Autodesk Inventor part; units mm, degrees
(part 8 of 13)
  line L3379 (11.7489, 33.1395) -> (11.9957, 33.1395) construction
  line L3380 (11.9957, 33.1395) -> (12.1959, 33.3398) construction
  line L3381 (12.1959, 33.3398) -> (12.1959, 33.5866) construction
  spline S1052 degree 3 poles (14.75, 33.5866) (14.75, 33.8334) (14.5498, 34.0334) (14.303, 34.0334) knots 0 0 0 0 1 1 1 1
  line L3382 (14.75, 33.5866) -> (14.75, 33.8334) construction
  line L3383 (14.75, 33.8334) -> (14.5498, 34.0334) construction
  line L3384 (14.5498, 34.0334) -> (14.303, 34.0334) construction
  spline S1053 degree 3 poles (14.303, 34.0334) (14.0562, 34.0334) (13.8561, 33.8334) (13.8561, 33.5866) knots 0 0 0 0 1 1 1 1
  line L3385 (14.303, 34.0334) -> (14.0562, 34.0334) construction
  line L3386 (14.0562, 34.0334) -> (13.8561, 33.8334) construction
  line L3387 (13.8561, 33.8334) -> (13.8561, 33.5866) construction
  spline S1054 degree 3 poles (13.8561, 33.5866) (13.8561, 33.3398) (14.0562, 33.1395) (14.303, 33.1395) knots 0 0 0 0 1 1 1 1
  line L3388 (13.8561, 33.5866) -> (13.8561, 33.3398) construction
  line L3389 (13.8561, 33.3398) -> (14.0562, 33.1395) construction
  line L3390 (14.0562, 33.1395) -> (14.303, 33.1395) construction
  spline S1055 degree 3 poles (14.303, 33.1395) (14.5498, 33.1395) (14.75, 33.3398) (14.75, 33.5866) knots 0 0 0 0 1 1 1 1
  line L3391 (14.303, 33.1395) -> (14.5498, 33.1395) construction
  line L3392 (14.5498, 33.1395) -> (14.75, 33.3398) construction
  line L3393 (14.75, 33.3398) -> (14.75, 33.5866) construction
  spline S1056 degree 3 poles (17.3041, 23.3701) (17.3041, 23.6169) (17.1039, 23.817) (16.8571, 23.817) knots 0 0 0 0 1 1 1 1
  line L3394 (17.3041, 23.3701) -> (17.3041, 23.6169) construction
  line L3395 (17.3041, 23.6169) -> (17.1039, 23.817) construction
  line L3396 (17.1039, 23.817) -> (16.8571, 23.817) construction
  spline S1057 degree 3 poles (16.8571, 23.817) (16.6103, 23.817) (16.4102, 23.6169) (16.4102, 23.3701) knots 0 0 0 0 1 1 1 1
  line L3397 (16.8571, 23.817) -> (16.6103, 23.817) construction
  line L3398 (16.6103, 23.817) -> (16.4102, 23.6169) construction
  line L3399 (16.4102, 23.6169) -> (16.4102, 23.3701) construction
  spline S1058 degree 3 poles (16.4102, 23.3701) (16.4102, 23.1233) (16.6103, 22.9231) (16.8571, 22.9231) knots 0 0 0 0 1 1 1 1
  line L3400 (16.4102, 23.3701) -> (16.4102, 23.1233) construction
  line L3401 (16.4102, 23.1233) -> (16.6103, 22.9231) construction
  line L3402 (16.6103, 22.9231) -> (16.8571, 22.9231) construction
  spline S1059 degree 3 poles (16.8571, 22.9231) (17.1039, 22.9231) (17.3041, 23.1233) (17.3041, 23.3701) knots 0 0 0 0 1 1 1 1
  line L3403 (16.8571, 22.9231) -> (17.1039, 22.9231) construction
  line L3404 (17.1039, 22.9231) -> (17.3041, 23.1233) construction
  line L3405 (17.3041, 23.1233) -> (17.3041, 23.3701) construction
  spline S1060 degree 3 poles (22.7955, 22.2718) (22.7955, 22.5186) (22.5952, 22.7188) (22.3485, 22.7188) knots 0 0 0 0 1 1 1 1
  line L3406 (22.7955, 22.2718) -> (22.7955, 22.5186) construction
  line L3407 (22.7955, 22.5186) -> (22.5952, 22.7188) construction
  line L3408 (22.5952, 22.7188) -> (22.3485, 22.7188) construction
  spline S1061 degree 3 poles (22.3485, 22.7188) (22.1017, 22.7188) (21.9014, 22.5186) (21.9014, 22.2718) knots 0 0 0 0 1 1 1 1
  line L3409 (22.3485, 22.7188) -> (22.1017, 22.7188) construction
  line L3410 (22.1017, 22.7188) -> (21.9014, 22.5186) construction
  line L3411 (21.9014, 22.5186) -> (21.9014, 22.2718) construction
  spline S1062 degree 3 poles (21.9014, 22.2718) (21.9014, 22.025) (22.1017, 21.8248) (22.3485, 21.8248) knots 0 0 0 0 1 1 1 1
  line L3412 (21.9014, 22.2718) -> (21.9014, 22.025) construction
  line L3413 (21.9014, 22.025) -> (22.1017, 21.8248) construction
  line L3414 (22.1017, 21.8248) -> (22.3485, 21.8248) construction
  spline S1063 degree 3 poles (22.3485, 21.8248) (22.5952, 21.8248) (22.7955, 22.025) (22.7955, 22.2718) knots 0 0 0 0 1 1 1 1
  line L3415 (22.3485, 21.8248) -> (22.5952, 21.8248) construction
  line L3416 (22.5952, 21.8248) -> (22.7955, 22.025) construction
  line L3417 (22.7955, 22.025) -> (22.7955, 22.2718) construction
  spline S1064 degree 3 poles (25.3496, 22.2718) (25.3496, 22.5186) (25.1494, 22.7188) (24.9026, 22.7188) knots 0 0 0 0 1 1 1 1
  line L3418 (25.3496, 22.2718) -> (25.3496, 22.5186) construction
  line L3419 (25.3496, 22.5186) -> (25.1494, 22.7188) construction
  line L3420 (25.1494, 22.7188) -> (24.9026, 22.7188) construction
  spline S1065 degree 3 poles (24.9026, 22.7188) (24.6558, 22.7188) (24.4555, 22.5186) (24.4555, 22.2718) knots 0 0 0 0 1 1 1 1
  line L3421 (24.9026, 22.7188) -> (24.6558, 22.7188) construction
  line L3422 (24.6558, 22.7188) -> (24.4555, 22.5186) construction
  line L3423 (24.4555, 22.5186) -> (24.4555, 22.2718) construction
  spline S1066 degree 3 poles (24.4555, 22.2718) (24.4555, 22.025) (24.6558, 21.8248) (24.9026, 21.8248) knots 0 0 0 0 1 1 1 1
  line L3424 (24.4555, 22.2718) -> (24.4555, 22.025) construction
  line L3425 (24.4555, 22.025) -> (24.6558, 21.8248) construction
  line L3426 (24.6558, 21.8248) -> (24.9026, 21.8248) construction
  spline S1067 degree 3 poles (24.9026, 21.8248) (25.1494, 21.8248) (25.3496, 22.025) (25.3496, 22.2718) knots 0 0 0 0 1 1 1 1
  line L3427 (24.9026, 21.8248) -> (25.1494, 21.8248) construction
  line L3428 (25.1494, 21.8248) -> (25.3496, 22.025) construction
  line L3429 (25.3496, 22.025) -> (25.3496, 22.2718) construction
  spline S1068 degree 3 poles (22.7955, 24.8259) (22.7955, 25.0727) (22.5952, 25.2729) (22.3485, 25.2729) knots 0 0 0 0 1 1 1 1
  line L3430 (22.7955, 24.8259) -> (22.7955, 25.0727) construction
  line L3431 (22.7955, 25.0727) -> (22.5952, 25.2729) construction
  line L3432 (22.5952, 25.2729) -> (22.3485, 25.2729) construction
  spline S1069 degree 3 poles (22.3485, 25.2729) (22.1017, 25.2729) (21.9014, 25.0727) (21.9014, 24.8259) knots 0 0 0 0 1 1 1 1
  line L3433 (22.3485, 25.2729) -> (22.1017, 25.2729) construction
  line L3434 (22.1017, 25.2729) -> (21.9014, 25.0727) construction
  line L3435 (21.9014, 25.0727) -> (21.9014, 24.8259) construction
  spline S1070 degree 3 poles (21.9014, 24.8259) (21.9014, 24.5792) (22.1017, 24.3789) (22.3485, 24.3789) knots 0 0 0 0 1 1 1 1
  line L3436 (21.9014, 24.8259) -> (21.9014, 24.5792) construction
  line L3437 (21.9014, 24.5792) -> (22.1017, 24.3789) construction
  line L3438 (22.1017, 24.3789) -> (22.3485, 24.3789) construction
  spline S1071 degree 3 poles (22.3485, 24.3789) (22.5952, 24.3789) (22.7955, 24.5792) (22.7955, 24.8259) knots 0 0 0 0 1 1 1 1
  line L3439 (22.3485, 24.3789) -> (22.5952, 24.3789) construction
  line L3440 (22.5952, 24.3789) -> (22.7955, 24.5792) construction
  line L3441 (22.7955, 24.5792) -> (22.7955, 24.8259) construction
  spline S1072 degree 3 poles (25.3496, 24.8259) (25.3496, 25.0727) (25.1494, 25.2729) (24.9026, 25.2729) knots 0 0 0 0 1 1 1 1
  line L3442 (25.3496, 24.8259) -> (25.3496, 25.0727) construction
  line L3443 (25.3496, 25.0727) -> (25.1494, 25.2729) construction
  line L3444 (25.1494, 25.2729) -> (24.9026, 25.2729) construction
  spline S1073 degree 3 poles (24.9026, 25.2729) (24.6558, 25.2729) (24.4555, 25.0727) (24.4555, 24.8259) knots 0 0 0 0 1 1 1 1
  line L3445 (24.9026, 25.2729) -> (24.6558, 25.2729) construction
  line L3446 (24.6558, 25.2729) -> (24.4555, 25.0727) construction
  line L3447 (24.4555, 25.0727) -> (24.4555, 24.8259) construction
  spline S1074 degree 3 poles (24.4555, 24.8259) (24.4555, 24.5792) (24.6558, 24.3789) (24.9026, 24.3789) knots 0 0 0 0 1 1 1 1
  line L3448 (24.4555, 24.8259) -> (24.4555, 24.5792) construction
  line L3449 (24.4555, 24.5792) -> (24.6558, 24.3789) construction
  line L3450 (24.6558, 24.3789) -> (24.9026, 24.3789) construction
  spline S1075 degree 3 poles (24.9026, 24.3789) (25.1494, 24.3789) (25.3496, 24.5792) (25.3496, 24.8259) knots 0 0 0 0 1 1 1 1
  line L3451 (24.9026, 24.3789) -> (25.1494, 24.3789) construction
  line L3452 (25.1494, 24.3789) -> (25.3496, 24.5792) construction
  line L3453 (25.3496, 24.5792) -> (25.3496, 24.8259) construction
  spline S1076 degree 3 poles (19.8582, 23.3701) (19.8582, 23.6169) (19.658, 23.817) (19.4112, 23.817) knots 0 0 0 0 1 1 1 1
  line L3454 (19.8582, 23.3701) -> (19.8582, 23.6169) construction
  line L3455 (19.8582, 23.6169) -> (19.658, 23.817) construction
  line L3456 (19.658, 23.817) -> (19.4112, 23.817) construction
  spline S1077 degree 3 poles (19.4112, 23.817) (19.1644, 23.817) (18.9643, 23.6169) (18.9643, 23.3701) knots 0 0 0 0 1 1 1 1
  line L3457 (19.4112, 23.817) -> (19.1644, 23.817) construction
  line L3458 (19.1644, 23.817) -> (18.9643, 23.6169) construction
  line L3459 (18.9643, 23.6169) -> (18.9643, 23.3701) construction
  spline S1078 degree 3 poles (18.9643, 23.3701) (18.9643, 23.1233) (19.1644, 22.9231) (19.4112, 22.9231) knots 0 0 0 0 1 1 1 1
  line L3460 (18.9643, 23.3701) -> (18.9643, 23.1233) construction
  line L3461 (18.9643, 23.1233) -> (19.1644, 22.9231) construction
  line L3462 (19.1644, 22.9231) -> (19.4112, 22.9231) construction
  spline S1079 degree 3 poles (19.4112, 22.9231) (19.658, 22.9231) (19.8582, 23.1233) (19.8582, 23.3701) knots 0 0 0 0 1 1 1 1
  line L3463 (19.4112, 22.9231) -> (19.658, 22.9231) construction
  line L3464 (19.658, 22.9231) -> (19.8582, 23.1233) construction
  line L3465 (19.8582, 23.1233) -> (19.8582, 23.3701) construction
  spline S1080 degree 3 poles (19.8582, 25.9242) (19.8582, 26.171) (19.658, 26.3711) (19.4112, 26.3711) knots 0 0 0 0 1 1 1 1
  line L3466 (19.8582, 25.9242) -> (19.8582, 26.171) construction
  line L3467 (19.8582, 26.171) -> (19.658, 26.3711) construction
  line L3468 (19.658, 26.3711) -> (19.4112, 26.3711) construction
  spline S1081 degree 3 poles (19.4112, 26.3711) (19.1644, 26.3711) (18.9643, 26.171) (18.9643, 25.9242) knots 0 0 0 0 1 1 1 1
  line L3469 (19.4112, 26.3711) -> (19.1644, 26.3711) construction
  line L3470 (19.1644, 26.3711) -> (18.9643, 26.171) construction
  line L3471 (18.9643, 26.171) -> (18.9643, 25.9242) construction
  spline S1082 degree 3 poles (18.9643, 25.9242) (18.9643, 25.6775) (19.1644, 25.4772) (19.4112, 25.4772) knots 0 0 0 0 1 1 1 1
  line L3472 (18.9643, 25.9242) -> (18.9643, 25.6775) construction
  line L3473 (18.9643, 25.6775) -> (19.1644, 25.4772) construction
  line L3474 (19.1644, 25.4772) -> (19.4112, 25.4772) construction
  spline S1083 degree 3 poles (19.4112, 25.4772) (19.658, 25.4772) (19.8582, 25.6775) (19.8582, 25.9242) knots 0 0 0 0 1 1 1 1
  line L3475 (19.4112, 25.4772) -> (19.658, 25.4772) construction
  line L3476 (19.658, 25.4772) -> (19.8582, 25.6775) construction
  line L3477 (19.8582, 25.6775) -> (19.8582, 25.9242) construction
  spline S1084 degree 3 poles (19.8582, 28.4784) (19.8582, 28.7251) (19.658, 28.9252) (19.4112, 28.9252) knots 0 0 0 0 1 1 1 1
  line L3478 (19.8582, 28.4784) -> (19.8582, 28.7251) construction
  line L3479 (19.8582, 28.7251) -> (19.658, 28.9252) construction
  line L3480 (19.658, 28.9252) -> (19.4112, 28.9252) construction
  spline S1085 degree 3 poles (19.4112, 28.9252) (19.1644, 28.9252) (18.9643, 28.7251) (18.9643, 28.4784) knots 0 0 0 0 1 1 1 1
  line L3481 (19.4112, 28.9252) -> (19.1644, 28.9252) construction
  line L3482 (19.1644, 28.9252) -> (18.9643, 28.7251) construction
  line L3483 (18.9643, 28.7251) -> (18.9643, 28.4784) construction
  spline S1086 degree 3 poles (18.9643, 28.4784) (18.9643, 28.2316) (19.1644, 28.0313) (19.4112, 28.0313) knots 0 0 0 0 1 1 1 1
  line L3484 (18.9643, 28.4784) -> (18.9643, 28.2316) construction
  line L3485 (18.9643, 28.2316) -> (19.1644, 28.0313) construction
  line L3486 (19.1644, 28.0313) -> (19.4112, 28.0313) construction
  spline S1087 degree 3 poles (19.4112, 28.0313) (19.658, 28.0313) (19.8582, 28.2316) (19.8582, 28.4784) knots 0 0 0 0 1 1 1 1
  line L3487 (19.4112, 28.0313) -> (19.658, 28.0313) construction
  line L3488 (19.658, 28.0313) -> (19.8582, 28.2316) construction
  line L3489 (19.8582, 28.2316) -> (19.8582, 28.4784) construction
  spline S1088 degree 3 poles (19.8582, 31.0325) (19.8582, 31.2793) (19.658, 31.4793) (19.4112, 31.4793) knots 0 0 0 0 1 1 1 1
  line L3490 (19.8582, 31.0325) -> (19.8582, 31.2793) construction
  line L3491 (19.8582, 31.2793) -> (19.658, 31.4793) construction
  line L3492 (19.658, 31.4793) -> (19.4112, 31.4793) construction
  spline S1089 degree 3 poles (19.4112, 31.4793) (19.1644, 31.4793) (18.9643, 31.2793) (18.9643, 31.0325) knots 0 0 0 0 1 1 1 1
  line L3493 (19.4112, 31.4793) -> (19.1644, 31.4793) construction
  line L3494 (19.1644, 31.4793) -> (18.9643, 31.2793) construction
  line L3495 (18.9643, 31.2793) -> (18.9643, 31.0325) construction
  spline S1090 degree 3 poles (18.9643, 31.0325) (18.9643, 30.7857) (19.1644, 30.5854) (19.4112, 30.5854) knots 0 0 0 0 1 1 1 1
  line L3496 (18.9643, 31.0325) -> (18.9643, 30.7857) construction
  line L3497 (18.9643, 30.7857) -> (19.1644, 30.5854) construction
  line L3498 (19.1644, 30.5854) -> (19.4112, 30.5854) construction
  spline S1091 degree 3 poles (19.4112, 30.5854) (19.658, 30.5854) (19.8582, 30.7857) (19.8582, 31.0325) knots 0 0 0 0 1 1 1 1
  line L3499 (19.4112, 30.5854) -> (19.658, 30.5854) construction
  line L3500 (19.658, 30.5854) -> (19.8582, 30.7857) construction
  line L3501 (19.8582, 30.7857) -> (19.8582, 31.0325) construction
  spline S1092 degree 3 poles (17.3041, 25.9242) (17.3041, 26.171) (17.1039, 26.3711) (16.8571, 26.3711) knots 0 0 0 0 1 1 1 1
  line L3502 (17.3041, 25.9242) -> (17.3041, 26.171) construction
  line L3503 (17.3041, 26.171) -> (17.1039, 26.3711) construction
  line L3504 (17.1039, 26.3711) -> (16.8571, 26.3711) construction
  spline S1093 degree 3 poles (16.8571, 26.3711) (16.6103, 26.3711) (16.4102, 26.171) (16.4102, 25.9242) knots 0 0 0 0 1 1 1 1
  line L3505 (16.8571, 26.3711) -> (16.6103, 26.3711) construction
  line L3506 (16.6103, 26.3711) -> (16.4102, 26.171) construction
  line L3507 (16.4102, 26.171) -> (16.4102, 25.9242) construction
  spline S1094 degree 3 poles (16.4102, 25.9242) (16.4102, 25.6775) (16.6103, 25.4772) (16.8571, 25.4772) knots 0 0 0 0 1 1 1 1
  line L3508 (16.4102, 25.9242) -> (16.4102, 25.6775) construction
  line L3509 (16.4102, 25.6775) -> (16.6103, 25.4772) construction
  line L3510 (16.6103, 25.4772) -> (16.8571, 25.4772) construction
  spline S1095 degree 3 poles (16.8571, 25.4772) (17.1039, 25.4772) (17.3041, 25.6775) (17.3041, 25.9242) knots 0 0 0 0 1 1 1 1
  line L3511 (16.8571, 25.4772) -> (17.1039, 25.4772) construction
  line L3512 (17.1039, 25.4772) -> (17.3041, 25.6775) construction
  line L3513 (17.3041, 25.6775) -> (17.3041, 25.9242) construction
  spline S1096 degree 3 poles (17.3041, 28.4784) (17.3041, 28.7251) (17.1039, 28.9252) (16.8571, 28.9252) knots 0 0 0 0 1 1 1 1
  line L3514 (17.3041, 28.4784) -> (17.3041, 28.7251) construction
  line L3515 (17.3041, 28.7251) -> (17.1039, 28.9252) construction
  line L3516 (17.1039, 28.9252) -> (16.8571, 28.9252) construction
  spline S1097 degree 3 poles (16.8571, 28.9252) (16.6103, 28.9252) (16.4102, 28.7251) (16.4102, 28.4784) knots 0 0 0 0 1 1 1 1
  line L3517 (16.8571, 28.9252) -> (16.6103, 28.9252) construction
  line L3518 (16.6103, 28.9252) -> (16.4102, 28.7251) construction
  line L3519 (16.4102, 28.7251) -> (16.4102, 28.4784) construction
  spline S1098 degree 3 poles (16.4102, 28.4784) (16.4102, 28.2316) (16.6103, 28.0313) (16.8571, 28.0313) knots 0 0 0 0 1 1 1 1
  line L3520 (16.4102, 28.4784) -> (16.4102, 28.2316) construction
  line L3521 (16.4102, 28.2316) -> (16.6103, 28.0313) construction
  line L3522 (16.6103, 28.0313) -> (16.8571, 28.0313) construction
  spline S1099 degree 3 poles (16.8571, 28.0313) (17.1039, 28.0313) (17.3041, 28.2316) (17.3041, 28.4784) knots 0 0 0 0 1 1 1 1
  line L3523 (16.8571, 28.0313) -> (17.1039, 28.0313) construction
  line L3524 (17.1039, 28.0313) -> (17.3041, 28.2316) construction
  line L3525 (17.3041, 28.2316) -> (17.3041, 28.4784) construction
  spline S1100 degree 3 poles (17.3041, 31.0325) (17.3041, 31.2793) (17.1039, 31.4793) (16.8571, 31.4793) knots 0 0 0 0 1 1 1 1
  line L3526 (17.3041, 31.0325) -> (17.3041, 31.2793) construction
  line L3527 (17.3041, 31.2793) -> (17.1039, 31.4793) construction
  line L3528 (17.1039, 31.4793) -> (16.8571, 31.4793) construction
  spline S1101 degree 3 poles (16.8571, 31.4793) (16.6103, 31.4793) (16.4102, 31.2793) (16.4102, 31.0325) knots 0 0 0 0 1 1 1 1
  line L3529 (16.8571, 31.4793) -> (16.6103, 31.4793) construction
  line L3530 (16.6103, 31.4793) -> (16.4102, 31.2793) construction
  line L3531 (16.4102, 31.2793) -> (16.4102, 31.0325) construction
  spline S1102 degree 3 poles (16.4102, 31.0325) (16.4102, 30.7857) (16.6103, 30.5854) (16.8571, 30.5854) knots 0 0 0 0 1 1 1 1
  line L3532 (16.4102, 31.0325) -> (16.4102, 30.7857) construction
  line L3533 (16.4102, 30.7857) -> (16.6103, 30.5854) construction
  line L3534 (16.6103, 30.5854) -> (16.8571, 30.5854) construction
  spline S1103 degree 3 poles (16.8571, 30.5854) (17.1039, 30.5854) (17.3041, 30.7857) (17.3041, 31.0325) knots 0 0 0 0 1 1 1 1
  line L3535 (16.8571, 30.5854) -> (17.1039, 30.5854) construction
  line L3536 (17.1039, 30.5854) -> (17.3041, 30.7857) construction
  line L3537 (17.3041, 30.7857) -> (17.3041, 31.0325) construction
  spline S1104 degree 3 poles (37.737, 33.5866) (37.737, 33.8334) (37.5369, 34.0334) (37.29, 34.0334) knots 0 0 0 0 1 1 1 1
  line L3538 (37.737, 33.5866) -> (37.737, 33.8334) construction
  line L3539 (37.737, 33.8334) -> (37.5369, 34.0334) construction
  line L3540 (37.5369, 34.0334) -> (37.29, 34.0334) construction
  spline S1105 degree 3 poles (37.29, 34.0334) (37.0431, 34.0334) (36.843, 33.8334) (36.843, 33.5866) knots 0 0 0 0 1 1 1 1
  line L3541 (37.29, 34.0334) -> (37.0431, 34.0334) construction
  line L3542 (37.0431, 34.0334) -> (36.843, 33.8334) construction
  line L3543 (36.843, 33.8334) -> (36.843, 33.5866) construction
  spline S1106 degree 3 poles (36.843, 33.5866) (36.843, 33.3398) (37.0431, 33.1395) (37.29, 33.1395) knots 0 0 0 0 1 1 1 1
  line L3544 (36.843, 33.5866) -> (36.843, 33.3398) construction
  line L3545 (36.843, 33.3398) -> (37.0431, 33.1395) construction
  line L3546 (37.0431, 33.1395) -> (37.29, 33.1395) construction
  spline S1107 degree 3 poles (37.29, 33.1395) (37.5369, 33.1395) (37.737, 33.3398) (37.737, 33.5866) knots 0 0 0 0 1 1 1 1
  line L3547 (37.29, 33.1395) -> (37.5369, 33.1395) construction
  line L3548 (37.5369, 33.1395) -> (37.737, 33.3398) construction
  line L3549 (37.737, 33.3398) -> (37.737, 33.5866) construction
  spline S1108 degree 3 poles (40.2911, 33.5866) (40.2911, 33.8334) (40.091, 34.0334) (39.8441, 34.0334) knots 0 0 0 0 1 1 1 1
  line L3550 (40.2911, 33.5866) -> (40.2911, 33.8334) construction
  line L3551 (40.2911, 33.8334) -> (40.091, 34.0334) construction
  line L3552 (40.091, 34.0334) -> (39.8441, 34.0334) construction
  spline S1109 degree 3 poles (39.8441, 34.0334) (39.5972, 34.0334) (39.3971, 33.8334) (39.3971, 33.5866) knots 0 0 0 0 1 1 1 1
  line L3553 (39.8441, 34.0334) -> (39.5972, 34.0334) construction
  line L3554 (39.5972, 34.0334) -> (39.3971, 33.8334) construction
  line L3555 (39.3971, 33.8334) -> (39.3971, 33.5866) construction
  spline S1110 degree 3 poles (39.3971, 33.5866) (39.3971, 33.3398) (39.5972, 33.1395) (39.8441, 33.1395) knots 0 0 0 0 1 1 1 1
  line L3556 (39.3971, 33.5866) -> (39.3971, 33.3398) construction
  line L3557 (39.3971, 33.3398) -> (39.5972, 33.1395) construction
  line L3558 (39.5972, 33.1395) -> (39.8441, 33.1395) construction
  spline S1111 degree 3 poles (39.8441, 33.1395) (40.091, 33.1395) (40.2911, 33.3398) (40.2911, 33.5866) knots 0 0 0 0 1 1 1 1
  line L3559 (39.8441, 33.1395) -> (40.091, 33.1395) construction
  line L3560 (40.091, 33.1395) -> (40.2911, 33.3398) construction
  line L3561 (40.2911, 33.3398) -> (40.2911, 33.5866) construction
  spline S1112 degree 3 poles (42.8452, 33.5866) (42.8452, 33.8334) (42.6451, 34.0334) (42.3982, 34.0334) knots 0 0 0 0 1 1 1 1
  line L3562 (42.8452, 33.5866) -> (42.8452, 33.8334) construction
  line L3563 (42.8452, 33.8334) -> (42.6451, 34.0334) construction
  line L3564 (42.6451, 34.0334) -> (42.3982, 34.0334) construction
  spline S1113 degree 3 poles (42.3982, 34.0334) (42.1513, 34.0334) (41.9512, 33.8334) (41.9512, 33.5866) knots 0 0 0 0 1 1 1 1
  line L3565 (42.3982, 34.0334) -> (42.1513, 34.0334) construction
  line L3566 (42.1513, 34.0334) -> (41.9512, 33.8334) construction
  line L3567 (41.9512, 33.8334) -> (41.9512, 33.5866) construction
  spline S1114 degree 3 poles (41.9512, 33.5866) (41.9512, 33.3398) (42.1513, 33.1395) (42.3982, 33.1395) knots 0 0 0 0 1 1 1 1
  line L3568 (41.9512, 33.5866) -> (41.9512, 33.3398) construction
  line L3569 (41.9512, 33.3398) -> (42.1513, 33.1395) construction
  line L3570 (42.1513, 33.1395) -> (42.3982, 33.1395) construction
  spline S1115 degree 3 poles (42.3982, 33.1395) (42.6451, 33.1395) (42.8452, 33.3398) (42.8452, 33.5866) knots 0 0 0 0 1 1 1 1
  line L3571 (42.3982, 33.1395) -> (42.6451, 33.1395) construction
  line L3572 (42.6451, 33.1395) -> (42.8452, 33.3398) construction
  line L3573 (42.8452, 33.3398) -> (42.8452, 33.5866) construction
  spline S1116 degree 3 poles (45.3993, 33.5866) (45.3993, 33.8334) (45.1992, 34.0334) (44.9523, 34.0334) knots 0 0 0 0 1 1 1 1
  line L3574 (45.3993, 33.5866) -> (45.3993, 33.8334) construction
  line L3575 (45.3993, 33.8334) -> (45.1992, 34.0334) construction
  line L3576 (45.1992, 34.0334) -> (44.9523, 34.0334) construction
  spline S1117 degree 3 poles (44.9523, 34.0334) (44.7054, 34.0334) (44.5054, 33.8334) (44.5054, 33.5866) knots 0 0 0 0 1 1 1 1
  line L3577 (44.9523, 34.0334) -> (44.7054, 34.0334) construction
  line L3578 (44.7054, 34.0334) -> (44.5054, 33.8334) construction
  line L3579 (44.5054, 33.8334) -> (44.5054, 33.5866) construction
  spline S1118 degree 3 poles (44.5054, 33.5866) (44.5054, 33.3398) (44.7054, 33.1395) (44.9523, 33.1395) knots 0 0 0 0 1 1 1 1
  line L3580 (44.5054, 33.5866) -> (44.5054, 33.3398) construction
  line L3581 (44.5054, 33.3398) -> (44.7054, 33.1395) construction
  line L3582 (44.7054, 33.1395) -> (44.9523, 33.1395) construction
  spline S1119 degree 3 poles (44.9523, 33.1395) (45.1992, 33.1395) (45.3993, 33.3398) (45.3993, 33.5866) knots 0 0 0 0 1 1 1 1
  line L3583 (44.9523, 33.1395) -> (45.1992, 33.1395) construction
  line L3584 (45.1992, 33.1395) -> (45.3993, 33.3398) construction
  line L3585 (45.3993, 33.3398) -> (45.3993, 33.5866) construction
  spline S1120 degree 3 poles (33.9058, 0.3832) (33.9058, 0.6299) (33.7056, 0.83) (33.4588, 0.83) knots 0 0 0 0 1 1 1 1
  line L3586 (33.9058, 0.3832) -> (33.9058, 0.6299) construction
  line L3587 (33.9058, 0.6299) -> (33.7056, 0.83) construction
  line L3588 (33.7056, 0.83) -> (33.4588, 0.83) construction
  spline S1121 degree 3 poles (33.4588, 0.83) (33.212, 0.83) (33.0119, 0.6299) (33.0119, 0.3832) knots 0 0 0 0 1 1 1 1
  line L3589 (33.4588, 0.83) -> (33.212, 0.83) construction
  line L3590 (33.212, 0.83) -> (33.0119, 0.6299) construction
  line L3591 (33.0119, 0.6299) -> (33.0119, 0.3832) construction
  spline S1122 degree 3 poles (33.0119, 0.3832) (33.0119, 0.1364) (33.212, -0.0639) (33.4588, -0.0639) knots 0 0 0 0 1 1 1 1
  line L3592 (33.0119, 0.3832) -> (33.0119, 0.1364) construction
  line L3593 (33.0119, 0.1364) -> (33.212, -0.0639) construction
  line L3594 (33.212, -0.0639) -> (33.4588, -0.0639) construction
  spline S1123 degree 3 poles (33.4588, -0.0639) (33.7056, -0.0639) (33.9058, 0.1364) (33.9058, 0.3832) knots 0 0 0 0 1 1 1 1
  line L3595 (33.4588, -0.0639) -> (33.7056, -0.0639) construction
  line L3596 (33.7056, -0.0639) -> (33.9058, 0.1364) construction
  line L3597 (33.9058, 0.1364) -> (33.9058, 0.3832) construction
  spline S1124 degree 3 poles (31.3517, 0.3832) (31.3517, 0.6299) (31.1515, 0.83) (30.9047, 0.83) knots 0 0 0 0 1 1 1 1
  line L3598 (31.3517, 0.3832) -> (31.3517, 0.6299) construction
  line L3599 (31.3517, 0.6299) -> (31.1515, 0.83) construction
  line L3600 (31.1515, 0.83) -> (30.9047, 0.83) construction
  spline S1125 degree 3 poles (30.9047, 0.83) (30.6579, 0.83) (30.4578, 0.6299) (30.4578, 0.3832) knots 0 0 0 0 1 1 1 1
  line L3601 (30.9047, 0.83) -> (30.6579, 0.83) construction
  line L3602 (30.6579, 0.83) -> (30.4578, 0.6299) construction
  line L3603 (30.4578, 0.6299) -> (30.4578, 0.3832) construction
  spline S1126 degree 3 poles (30.4578, 0.3832) (30.4578, 0.1364) (30.6579, -0.0639) (30.9047, -0.0639) knots 0 0 0 0 1 1 1 1
  line L3604 (30.4578, 0.3832) -> (30.4578, 0.1364) construction
  line L3605 (30.4578, 0.1364) -> (30.6579, -0.0639) construction
  line L3606 (30.6579, -0.0639) -> (30.9047, -0.0639) construction
  spline S1127 degree 3 poles (30.9047, -0.0639) (31.1515, -0.0639) (31.3517, 0.1364) (31.3517, 0.3832) knots 0 0 0 0 1 1 1 1
  line L3607 (30.9047, -0.0639) -> (31.1515, -0.0639) construction
  line L3608 (31.1515, -0.0639) -> (31.3517, 0.1364) construction
  line L3609 (31.3517, 0.1364) -> (31.3517, 0.3832) construction
  spline S1128 degree 3 poles (28.7976, 0.3832) (28.7976, 0.6299) (28.5974, 0.83) (28.3506, 0.83) knots 0 0 0 0 1 1 1 1
  line L3610 (28.7976, 0.3832) -> (28.7976, 0.6299) construction
  line L3611 (28.7976, 0.6299) -> (28.5974, 0.83) construction
  line L3612 (28.5974, 0.83) -> (28.3506, 0.83) construction
  spline S1129 degree 3 poles (28.3506, 0.83) (28.1038, 0.83) (27.9037, 0.6299) (27.9037, 0.3832) knots 0 0 0 0 1 1 1 1
  line L3613 (28.3506, 0.83) -> (28.1038, 0.83) construction
  line L3614 (28.1038, 0.83) -> (27.9037, 0.6299) construction
  line L3615 (27.9037, 0.6299) -> (27.9037, 0.3832) construction
  spline S1130 degree 3 poles (27.9037, 0.3832) (27.9037, 0.1364) (28.1038, -0.0639) (28.3506, -0.0639) knots 0 0 0 0 1 1 1 1
  line L3616 (27.9037, 0.3832) -> (27.9037, 0.1364) construction
  line L3617 (27.9037, 0.1364) -> (28.1038, -0.0639) construction
  line L3618 (28.1038, -0.0639) -> (28.3506, -0.0639) construction
  spline S1131 degree 3 poles (28.3506, -0.0639) (28.5974, -0.0639) (28.7976, 0.1364) (28.7976, 0.3832) knots 0 0 0 0 1 1 1 1
  line L3619 (28.3506, -0.0639) -> (28.5974, -0.0639) construction
  line L3620 (28.5974, -0.0639) -> (28.7976, 0.1364) construction
  line L3621 (28.7976, 0.1364) -> (28.7976, 0.3832) construction
  spline S1132 degree 3 poles (42.8452, 0.3832) (42.8452, 0.6299) (42.6451, 0.83) (42.3982, 0.83) knots 0 0 0 0 1 1 1 1
  line L3622 (42.8452, 0.3832) -> (42.8452, 0.6299) construction
  line L3623 (42.8452, 0.6299) -> (42.6451, 0.83) construction
  line L3624 (42.6451, 0.83) -> (42.3982, 0.83) construction
  spline S1133 degree 3 poles (42.3982, 0.83) (42.1513, 0.83) (41.9512, 0.6299) (41.9512, 0.3832) knots 0 0 0 0 1 1 1 1
  line L3625 (42.3982, 0.83) -> (42.1513, 0.83) construction
  line L3626 (42.1513, 0.83) -> (41.9512, 0.6299) construction
  line L3627 (41.9512, 0.6299) -> (41.9512, 0.3832) construction
  spline S1134 degree 3 poles (41.9512, 0.3832) (41.9512, 0.1364) (42.1513, -0.0639) (42.3982, -0.0639) knots 0 0 0 0 1 1 1 1
  line L3628 (41.9512, 0.3832) -> (41.9512, 0.1364) construction
  line L3629 (41.9512, 0.1364) -> (42.1513, -0.0639) construction
  line L3630 (42.1513, -0.0639) -> (42.3982, -0.0639) construction
  spline S1135 degree 3 poles (42.3982, -0.0639) (42.6451, -0.0639) (42.8452, 0.1364) (42.8452, 0.3832) knots 0 0 0 0 1 1 1 1
  line L3631 (42.3982, -0.0639) -> (42.6451, -0.0639) construction
  line L3632 (42.6451, -0.0639) -> (42.8452, 0.1364) construction
  line L3633 (42.8452, 0.1364) -> (42.8452, 0.3832) construction
  spline S1136 degree 3 poles (35.1829, 2.9373) (35.1829, 3.1841) (34.9826, 3.3841) (34.7358, 3.3841) knots 0 0 0 0 1 1 1 1
  line L3634 (35.1829, 2.9373) -> (35.1829, 3.1841) construction
  line L3635 (35.1829, 3.1841) -> (34.9826, 3.3841) construction
  line L3636 (34.9826, 3.3841) -> (34.7358, 3.3841) construction
  spline S1137 degree 3 poles (34.7358, 3.3841) (34.4891, 3.3841) (34.289, 3.1841) (34.289, 2.9373) knots 0 0 0 0 1 1 1 1
  line L3637 (34.7358, 3.3841) -> (34.4891, 3.3841) construction
  line L3638 (34.4891, 3.3841) -> (34.289, 3.1841) construction
  line L3639 (34.289, 3.1841) -> (34.289, 2.9373) construction
  spline S1138 degree 3 poles (34.289, 2.9373) (34.289, 2.6905) (34.4891, 2.4902) (34.7358, 2.4902) knots 0 0 0 0 1 1 1 1
  line L3640 (34.289, 2.9373) -> (34.289, 2.6905) construction
  line L3641 (34.289, 2.6905) -> (34.4891, 2.4902) construction
  line L3642 (34.4891, 2.4902) -> (34.7358, 2.4902) construction
  spline S1139 degree 3 poles (34.7358, 2.4902) (34.9826, 2.4902) (35.1829, 2.6905) (35.1829, 2.9373) knots 0 0 0 0 1 1 1 1
  line L3643 (34.7358, 2.4902) -> (34.9826, 2.4902) construction
  line L3644 (34.9826, 2.4902) -> (35.1829, 2.6905) construction
  line L3645 (35.1829, 2.6905) -> (35.1829, 2.9373) construction
  spline S1140 degree 3 poles (35.1829, 5.4914) (35.1829, 5.7382) (34.9826, 5.9382) (34.7358, 5.9382) knots 0 0 0 0 1 1 1 1
  line L3646 (35.1829, 5.4914) -> (35.1829, 5.7382) construction
  line L3647 (35.1829, 5.7382) -> (34.9826, 5.9382) construction
  line L3648 (34.9826, 5.9382) -> (34.7358, 5.9382) construction
  spline S1141 degree 3 poles (34.7358, 5.9382) (34.4891, 5.9382) (34.289, 5.7382) (34.289, 5.4914) knots 0 0 0 0 1 1 1 1
  line L3649 (34.7358, 5.9382) -> (34.4891, 5.9382) construction
  line L3650 (34.4891, 5.9382) -> (34.289, 5.7382) construction
  line L3651 (34.289, 5.7382) -> (34.289, 5.4914) construction
  spline S1142 degree 3 poles (34.289, 5.4914) (34.289, 5.2446) (34.4891, 5.0443) (34.7358, 5.0443) knots 0 0 0 0 1 1 1 1
  line L3652 (34.289, 5.4914) -> (34.289, 5.2446) construction
  line L3653 (34.289, 5.2446) -> (34.4891, 5.0443) construction
  line L3654 (34.4891, 5.0443) -> (34.7358, 5.0443) construction
  spline S1143 degree 3 poles (34.7358, 5.0443) (34.9826, 5.0443) (35.1829, 5.2446) (35.1829, 5.4914) knots 0 0 0 0 1 1 1 1
  line L3655 (34.7358, 5.0443) -> (34.9826, 5.0443) construction
  line L3656 (34.9826, 5.0443) -> (35.1829, 5.2446) construction
  line L3657 (35.1829, 5.2446) -> (35.1829, 5.4914) construction
  spline S1144 degree 3 poles (37.737, 5.4914) (37.737, 5.7382) (37.5369, 5.9382) (37.29, 5.9382) knots 0 0 0 0 1 1 1 1
  line L3658 (37.737, 5.4914) -> (37.737, 5.7382) construction
  line L3659 (37.737, 5.7382) -> (37.5369, 5.9382) construction
  line L3660 (37.5369, 5.9382) -> (37.29, 5.9382) construction
  spline S1145 degree 3 poles (37.29, 5.9382) (37.0431, 5.9382) (36.843, 5.7382) (36.843, 5.4914) knots 0 0 0 0 1 1 1 1
  line L3661 (37.29, 5.9382) -> (37.0431, 5.9382) construction
  line L3662 (37.0431, 5.9382) -> (36.843, 5.7382) construction
  line L3663 (36.843, 5.7382) -> (36.843, 5.4914) construction
  spline S1146 degree 3 poles (36.843, 5.4914) (36.843, 5.2446) (37.0431, 5.0443) (37.29, 5.0443) knots 0 0 0 0 1 1 1 1
  line L3664 (36.843, 5.4914) -> (36.843, 5.2446) construction
  line L3665 (36.843, 5.2446) -> (37.0431, 5.0443) construction
  line L3666 (37.0431, 5.0443) -> (37.29, 5.0443) construction
  spline S1147 degree 3 poles (37.29, 5.0443) (37.5369, 5.0443) (37.737, 5.2446) (37.737, 5.4914) knots 0 0 0 0 1 1 1 1
  line L3667 (37.29, 5.0443) -> (37.5369, 5.0443) construction
  line L3668 (37.5369, 5.0443) -> (37.737, 5.2446) construction
  line L3669 (37.737, 5.2446) -> (37.737, 5.4914) construction
  spline S1148 degree 3 poles (37.737, 0.3832) (37.737, 0.6299) (37.5369, 0.83) (37.29, 0.83) knots 0 0 0 0 1 1 1 1
  line L3670 (37.737, 0.3832) -> (37.737, 0.6299) construction
  line L3671 (37.737, 0.6299) -> (37.5369, 0.83) construction
  line L3672 (37.5369, 0.83) -> (37.29, 0.83) construction
  spline S1149 degree 3 poles (37.29, 0.83) (37.0431, 0.83) (36.843, 0.6299) (36.843, 0.3832) knots 0 0 0 0 1 1 1 1
  line L3673 (37.29, 0.83) -> (37.0431, 0.83) construction
  line L3674 (37.0431, 0.83) -> (36.843, 0.6299) construction
  line L3675 (36.843, 0.6299) -> (36.843, 0.3832) construction
  spline S1150 degree 3 poles (36.843, 0.3832) (36.843, 0.1364) (37.0431, -0.0639) (37.29, -0.0639) knots 0 0 0 0 1 1 1 1
  line L3676 (36.843, 0.3832) -> (36.843, 0.1364) construction
  line L3677 (36.843, 0.1364) -> (37.0431, -0.0639) construction
  line L3678 (37.0431, -0.0639) -> (37.29, -0.0639) construction
  spline S1151 degree 3 poles (37.29, -0.0639) (37.5369, -0.0639) (37.737, 0.1364) (37.737, 0.3832) knots 0 0 0 0 1 1 1 1
  line L3679 (37.29, -0.0639) -> (37.5369, -0.0639) construction
  line L3680 (37.5369, -0.0639) -> (37.737, 0.1364) construction
  line L3681 (37.737, 0.1364) -> (37.737, 0.3832) construction
  spline S1152 degree 3 poles (40.2911, 0.3832) (40.2911, 0.6299) (40.091, 0.83) (39.8441, 0.83) knots 0 0 0 0 1 1 1 1
  line L3682 (40.2911, 0.3832) -> (40.2911, 0.6299) construction
  line L3683 (40.2911, 0.6299) -> (40.091, 0.83) construction
  line L3684 (40.091, 0.83) -> (39.8441, 0.83) construction
  spline S1153 degree 3 poles (39.8441, 0.83) (39.5972, 0.83) (39.3971, 0.6299) (39.3971, 0.3832) knots 0 0 0 0 1 1 1 1
  line L3685 (39.8441, 0.83) -> (39.5972, 0.83) construction
  line L3686 (39.5972, 0.83) -> (39.3971, 0.6299) construction
  line L3687 (39.3971, 0.6299) -> (39.3971, 0.3832) construction
  spline S1154 degree 3 poles (39.3971, 0.3832) (39.3971, 0.1364) (39.5972, -0.0639) (39.8441, -0.0639) knots 0 0 0 0 1 1 1 1
  line L3688 (39.3971, 0.3832) -> (39.3971, 0.1364) construction
  line L3689 (39.3971, 0.1364) -> (39.5972, -0.0639) construction
  line L3690 (39.5972, -0.0639) -> (39.8441, -0.0639) construction
  spline S1155 degree 3 poles (39.8441, -0.0639) (40.091, -0.0639) (40.2911, 0.1364) (40.2911, 0.3832) knots 0 0 0 0 1 1 1 1
  line L3691 (39.8441, -0.0639) -> (40.091, -0.0639) construction
  line L3692 (40.091, -0.0639) -> (40.2911, 0.1364) construction
  line L3693 (40.2911, 0.1364) -> (40.2911, 0.3832) construction
  spline S1156 degree 3 poles (37.737, 2.9373) (37.737, 3.1841) (37.5369, 3.3841) (37.29, 3.3841) knots 0 0 0 0 1 1 1 1
  line L3694 (37.737, 2.9373) -> (37.737, 3.1841) construction
  line L3695 (37.737, 3.1841) -> (37.5369, 3.3841) construction
  line L3696 (37.5369, 3.3841) -> (37.29, 3.3841) construction
  spline S1157 degree 3 poles (37.29, 3.3841) (37.0431, 3.3841) (36.843, 3.1841) (36.843, 2.9373) knots 0 0 0 0 1 1 1 1
  line L3697 (37.29, 3.3841) -> (37.0431, 3.3841) construction
  line L3698 (37.0431, 3.3841) -> (36.843, 3.1841) construction
  line L3699 (36.843, 3.1841) -> (36.843, 2.9373) construction
  spline S1158 degree 3 poles (36.843, 2.9373) (36.843, 2.6905) (37.0431, 2.4902) (37.29, 2.4902) knots 0 0 0 0 1 1 1 1
  line L3700 (36.843, 2.9373) -> (36.843, 2.6905) construction
  line L3701 (36.843, 2.6905) -> (37.0431, 2.4902) construction
  line L3702 (37.0431, 2.4902) -> (37.29, 2.4902) construction
  spline S1159 degree 3 poles (37.29, 2.4902) (37.5369, 2.4902) (37.737, 2.6905) (37.737, 2.9373) knots 0 0 0 0 1 1 1 1
  line L3703 (37.29, 2.4902) -> (37.5369, 2.4902) construction
  line L3704 (37.5369, 2.4902) -> (37.737, 2.6905) construction
  line L3705 (37.737, 2.6905) -> (37.737, 2.9373) construction
  spline S1160 degree 3 poles (35.1829, 8.0455) (35.1829, 8.2923) (34.9826, 8.4923) (34.7358, 8.4923) knots 0 0 0 0 1 1 1 1
  line L3706 (35.1829, 8.0455) -> (35.1829, 8.2923) construction
  line L3707 (35.1829, 8.2923) -> (34.9826, 8.4923) construction
  line L3708 (34.9826, 8.4923) -> (34.7358, 8.4923) construction
  spline S1161 degree 3 poles (34.7358, 8.4923) (34.4891, 8.4923) (34.289, 8.2923) (34.289, 8.0455) knots 0 0 0 0 1 1 1 1
  line L3709 (34.7358, 8.4923) -> (34.4891, 8.4923) construction
  line L3710 (34.4891, 8.4923) -> (34.289, 8.2923) construction
  line L3711 (34.289, 8.2923) -> (34.289, 8.0455) construction
  spline S1162 degree 3 poles (34.289, 8.0455) (34.289, 7.7987) (34.4891, 7.5984) (34.7358, 7.5984) knots 0 0 0 0 1 1 1 1
  line L3712 (34.289, 8.0455) -> (34.289, 7.7987) construction
  line L3713 (34.289, 7.7987) -> (34.4891, 7.5984) construction
  line L3714 (34.4891, 7.5984) -> (34.7358, 7.5984) construction
  spline S1163 degree 3 poles (34.7358, 7.5984) (34.9826, 7.5984) (35.1829, 7.7987) (35.1829, 8.0455) knots 0 0 0 0 1 1 1 1
  line L3715 (34.7358, 7.5984) -> (34.9826, 7.5984) construction
  line L3716 (34.9826, 7.5984) -> (35.1829, 7.7987) construction
  line L3717 (35.1829, 7.7987) -> (35.1829, 8.0455) construction
  spline S1164 degree 3 poles (37.737, 8.0455) (37.737, 8.2923) (37.5369, 8.4923) (37.29, 8.4923) knots 0 0 0 0 1 1 1 1
  line L3718 (37.737, 8.0455) -> (37.737, 8.2923) construction
  line L3719 (37.737, 8.2923) -> (37.5369, 8.4923) construction
  line L3720 (37.5369, 8.4923) -> (37.29, 8.4923) construction
  spline S1165 degree 3 poles (37.29, 8.4923) (37.0431, 8.4923) (36.843, 8.2923) (36.843, 8.0455) knots 0 0 0 0 1 1 1 1
  line L3721 (37.29, 8.4923) -> (37.0431, 8.4923) construction
  line L3722 (37.0431, 8.4923) -> (36.843, 8.2923) construction
  line L3723 (36.843, 8.2923) -> (36.843, 8.0455) construction
  spline S1166 degree 3 poles (36.843, 8.0455) (36.843, 7.7987) (37.0431, 7.5984) (37.29, 7.5984) knots 0 0 0 0 1 1 1 1
  line L3724 (36.843, 8.0455) -> (36.843, 7.7987) construction
  line L3725 (36.843, 7.7987) -> (37.0431, 7.5984) construction
  line L3726 (37.0431, 7.5984) -> (37.29, 7.5984) construction
  spline S1167 degree 3 poles (37.29, 7.5984) (37.5369, 7.5984) (37.737, 7.7987) (37.737, 8.0455) knots 0 0 0 0 1 1 1 1
  line L3727 (37.29, 7.5984) -> (37.5369, 7.5984) construction
  line L3728 (37.5369, 7.5984) -> (37.737, 7.7987) construction
  line L3729 (37.737, 7.7987) -> (37.737, 8.0455) construction
  spline S1168 degree 3 poles (35.1829, 10.5996) (35.1829, 10.8464) (34.9826, 11.0465) (34.7358, 11.0465) knots 0 0 0 0 1 1 1 1
  line L3730 (35.1829, 10.5996) -> (35.1829, 10.8464) construction
  line L3731 (35.1829, 10.8464) -> (34.9826, 11.0465) construction
  line L3732 (34.9826, 11.0465) -> (34.7358, 11.0465) construction
  spline S1169 degree 3 poles (34.7358, 11.0465) (34.4891, 11.0465) (34.289, 10.8464) (34.289, 10.5996) knots 0 0 0 0 1 1 1 1
  line L3733 (34.7358, 11.0465) -> (34.4891, 11.0465) construction
  line L3734 (34.4891, 11.0465) -> (34.289, 10.8464) construction
  line L3735 (34.289, 10.8464) -> (34.289, 10.5996) construction
  spline S1170 degree 3 poles (34.289, 10.5996) (34.289, 10.3528) (34.4891, 10.1525) (34.7358, 10.1525) knots 0 0 0 0 1 1 1 1
  line L3736 (34.289, 10.5996) -> (34.289, 10.3528) construction
  line L3737 (34.289, 10.3528) -> (34.4891, 10.1525) construction
  line L3738 (34.4891, 10.1525) -> (34.7358, 10.1525) construction
  spline S1171 degree 3 poles (34.7358, 10.1525) (34.9826, 10.1525) (35.1829, 10.3528) (35.1829, 10.5996) knots 0 0 0 0 1 1 1 1
  line L3739 (34.7358, 10.1525) -> (34.9826, 10.1525) construction
  line L3740 (34.9826, 10.1525) -> (35.1829, 10.3528) construction
  line L3741 (35.1829, 10.3528) -> (35.1829, 10.5996) construction
  spline S1172 degree 3 poles (37.737, 10.5996) (37.737, 10.8464) (37.5369, 11.0465) (37.29, 11.0465) knots 0 0 0 0 1 1 1 1
  line L3742 (37.737, 10.5996) -> (37.737, 10.8464) construction
  line L3743 (37.737, 10.8464) -> (37.5369, 11.0465) construction
  line L3744 (37.5369, 11.0465) -> (37.29, 11.0465) construction
  spline S1173 degree 3 poles (37.29, 11.0465) (37.0431, 11.0465) (36.843, 10.8464) (36.843, 10.5996) knots 0 0 0 0 1 1 1 1
  line L3745 (37.29, 11.0465) -> (37.0431, 11.0465) construction
  line L3746 (37.0431, 11.0465) -> (36.843, 10.8464) construction
  line L3747 (36.843, 10.8464) -> (36.843, 10.5996) construction
  spline S1174 degree 3 poles (36.843, 10.5996) (36.843, 10.3528) (37.0431, 10.1525) (37.29, 10.1525) knots 0 0 0 0 1 1 1 1
  line L3748 (36.843, 10.5996) -> (36.843, 10.3528) construction
  line L3749 (36.843, 10.3528) -> (37.0431, 10.1525) construction
  line L3750 (37.0431, 10.1525) -> (37.29, 10.1525) construction
  spline S1175 degree 3 poles (37.29, 10.1525) (37.5369, 10.1525) (37.737, 10.3528) (37.737, 10.5996) knots 0 0 0 0 1 1 1 1
  line L3751 (37.29, 10.1525) -> (37.5369, 10.1525) construction
  line L3752 (37.5369, 10.1525) -> (37.737, 10.3528) construction
  line L3753 (37.737, 10.3528) -> (37.737, 10.5996) construction
  spline S1176 degree 3 poles (35.1829, 13.1537) (35.1829, 13.4005) (34.9826, 13.6006) (34.7358, 13.6006) knots 0 0 0 0 1 1 1 1
  line L3754 (35.1829, 13.1537) -> (35.1829, 13.4005) construction
  line L3755 (35.1829, 13.4005) -> (34.9826, 13.6006) construction
  line L3756 (34.9826, 13.6006) -> (34.7358, 13.6006) construction
  spline S1177 degree 3 poles (34.7358, 13.6006) (34.4891, 13.6006) (34.289, 13.4005) (34.289, 13.1537) knots 0 0 0 0 1 1 1 1
  line L3757 (34.7358, 13.6006) -> (34.4891, 13.6006) construction
  line L3758 (34.4891, 13.6006) -> (34.289, 13.4005) construction
  line L3759 (34.289, 13.4005) -> (34.289, 13.1537) construction
  spline S1178 degree 3 poles (34.289, 13.1537) (34.289, 12.9069) (34.4891, 12.7067) (34.7358, 12.7067) knots 0 0 0 0 1 1 1 1
  line L3760 (34.289, 13.1537) -> (34.289, 12.9069) construction
  line L3761 (34.289, 12.9069) -> (34.4891, 12.7067) construction
  line L3762 (34.4891, 12.7067) -> (34.7358, 12.7067) construction
  spline S1179 degree 3 poles (34.7358, 12.7067) (34.9826, 12.7067) (35.1829, 12.9069) (35.1829, 13.1537) knots 0 0 0 0 1 1 1 1
  line L3763 (34.7358, 12.7067) -> (34.9826, 12.7067) construction
  line L3764 (34.9826, 12.7067) -> (35.1829, 12.9069) construction
  line L3765 (35.1829, 12.9069) -> (35.1829, 13.1537) construction
  spline S1180 degree 3 poles (37.737, 13.1537) (37.737, 13.4005) (37.5369, 13.6006) (37.29, 13.6006) knots 0 0 0 0 1 1 1 1
  line L3766 (37.737, 13.1537) -> (37.737, 13.4005) construction
  line L3767 (37.737, 13.4005) -> (37.5369, 13.6006) construction
  line L3768 (37.5369, 13.6006) -> (37.29, 13.6006) construction
  spline S1181 degree 3 poles (37.29, 13.6006) (37.0431, 13.6006) (36.843, 13.4005) (36.843, 13.1537) knots 0 0 0 0 1 1 1 1
  line L3769 (37.29, 13.6006) -> (37.0431, 13.6006) construction
  line L3770 (37.0431, 13.6006) -> (36.843, 13.4005) construction
  line L3771 (36.843, 13.4005) -> (36.843, 13.1537) construction
  spline S1182 degree 3 poles (36.843, 13.1537) (36.843, 12.9069) (37.0431, 12.7067) (37.29, 12.7067) knots 0 0 0 0 1 1 1 1
  line L3772 (36.843, 13.1537) -> (36.843, 12.9069) construction
  line L3773 (36.843, 12.9069) -> (37.0431, 12.7067) construction
  line L3774 (37.0431, 12.7067) -> (37.29, 12.7067) construction
  spline S1183 degree 3 poles (37.29, 12.7067) (37.5369, 12.7067) (37.737, 12.9069) (37.737, 13.1537) knots 0 0 0 0 1 1 1 1
  line L3775 (37.29, 12.7067) -> (37.5369, 12.7067) construction
  line L3776 (37.5369, 12.7067) -> (37.737, 12.9069) construction
  line L3777 (37.737, 12.9069) -> (37.737, 13.1537) construction
  spline S1184 degree 3 poles (35.1829, 15.7078) (35.1829, 15.9546) (34.9826, 16.1547) (34.7358, 16.1547) knots 0 0 0 0 1 1 1 1
  line L3778 (35.1829, 15.7078) -> (35.1829, 15.9546) construction
  line L3779 (35.1829, 15.9546) -> (34.9826, 16.1547) construction
  line L3780 (34.9826, 16.1547) -> (34.7358, 16.1547) construction
  spline S1185 degree 3 poles (34.7358, 16.1547) (34.4891, 16.1547) (34.289, 15.9546) (34.289, 15.7078) knots 0 0 0 0 1 1 1 1
  line L3781 (34.7358, 16.1547) -> (34.4891, 16.1547) construction
  line L3782 (34.4891, 16.1547) -> (34.289, 15.9546) construction
  line L3783 (34.289, 15.9546) -> (34.289, 15.7078) construction
  spline S1186 degree 3 poles (34.289, 15.7078) (34.289, 15.461) (34.4891, 15.2608) (34.7358, 15.2608) knots 0 0 0 0 1 1 1 1
  line L3784 (34.289, 15.7078) -> (34.289, 15.461) construction
  line L3785 (34.289, 15.461) -> (34.4891, 15.2608) construction
  line L3786 (34.4891, 15.2608) -> (34.7358, 15.2608) construction
  spline S1187 degree 3 poles (34.7358, 15.2608) (34.9826, 15.2608) (35.1829, 15.461) (35.1829, 15.7078) knots 0 0 0 0 1 1 1 1
  line L3787 (34.7358, 15.2608) -> (34.9826, 15.2608) construction
  line L3788 (34.9826, 15.2608) -> (35.1829, 15.461) construction
  line L3789 (35.1829, 15.461) -> (35.1829, 15.7078) construction
  spline S1188 degree 3 poles (37.737, 15.7078) (37.737, 15.9546) (37.5369, 16.1547) (37.29, 16.1547) knots 0 0 0 0 1 1 1 1
  line L3790 (37.737, 15.7078) -> (37.737, 15.9546) construction
  line L3791 (37.737, 15.9546) -> (37.5369, 16.1547) construction
  line L3792 (37.5369, 16.1547) -> (37.29, 16.1547) construction
  spline S1189 degree 3 poles (37.29, 16.1547) (37.0431, 16.1547) (36.843, 15.9546) (36.843, 15.7078) knots 0 0 0 0 1 1 1 1
  line L3793 (37.29, 16.1547) -> (37.0431, 16.1547) construction
  line L3794 (37.0431, 16.1547) -> (36.843, 15.9546) construction
  line L3795 (36.843, 15.9546) -> (36.843, 15.7078) construction
  spline S1190 degree 3 poles (36.843, 15.7078) (36.843, 15.461) (37.0431, 15.2608) (37.29, 15.2608) knots 0 0 0 0 1 1 1 1
  line L3796 (36.843, 15.7078) -> (36.843, 15.461) construction
  line L3797 (36.843, 15.461) -> (37.0431, 15.2608) construction
  line L3798 (37.0431, 15.2608) -> (37.29, 15.2608) construction
  spline S1191 degree 3 poles (37.29, 15.2608) (37.5369, 15.2608) (37.737, 15.461) (37.737, 15.7078) knots 0 0 0 0 1 1 1 1
  line L3799 (37.29, 15.2608) -> (37.5369, 15.2608) construction
  line L3800 (37.5369, 15.2608) -> (37.737, 15.461) construction
  line L3801 (37.737, 15.461) -> (37.737, 15.7078) construction
  spline S1192 degree 3 poles (35.1829, 18.2619) (35.1829, 18.5087) (34.9826, 18.7088) (34.7358, 18.7088) knots 0 0 0 0 1 1 1 1
  line L3802 (35.1829, 18.2619) -> (35.1829, 18.5087) construction
  line L3803 (35.1829, 18.5087) -> (34.9826, 18.7088) construction
  line L3804 (34.9826, 18.7088) -> (34.7358, 18.7088) construction
  spline S1193 degree 3 poles (34.7358, 18.7088) (34.4891, 18.7088) (34.289, 18.5087) (34.289, 18.2619) knots 0 0 0 0 1 1 1 1
  line L3805 (34.7358, 18.7088) -> (34.4891, 18.7088) construction
  line L3806 (34.4891, 18.7088) -> (34.289, 18.5087) construction
  line L3807 (34.289, 18.5087) -> (34.289, 18.2619) construction
  spline S1194 degree 3 poles (34.289, 18.2619) (34.289, 18.0151) (34.4891, 17.8149) (34.7358, 17.8149) knots 0 0 0 0 1 1 1 1
  line L3808 (34.289, 18.2619) -> (34.289, 18.0151) construction
  line L3809 (34.289, 18.0151) -> (34.4891, 17.8149) construction
  line L3810 (34.4891, 17.8149) -> (34.7358, 17.8149) construction
  spline S1195 degree 3 poles (34.7358, 17.8149) (34.9826, 17.8149) (35.1829, 18.0151) (35.1829, 18.2619) knots 0 0 0 0 1 1 1 1
  line L3811 (34.7358, 17.8149) -> (34.9826, 17.8149) construction
  line L3812 (34.9826, 17.8149) -> (35.1829, 18.0151) construction
  line L3813 (35.1829, 18.0151) -> (35.1829, 18.2619) construction
  spline S1196 degree 3 poles (37.737, 18.2619) (37.737, 18.5087) (37.5369, 18.7088) (37.29, 18.7088) knots 0 0 0 0 1 1 1 1
  line L3814 (37.737, 18.2619) -> (37.737, 18.5087) construction
  line L3815 (37.737, 18.5087) -> (37.5369, 18.7088) construction
  line L3816 (37.5369, 18.7088) -> (37.29, 18.7088) construction
  spline S1197 degree 3 poles (37.29, 18.7088) (37.0431, 18.7088) (36.843, 18.5087) (36.843, 18.2619) knots 0 0 0 0 1 1 1 1
  line L3817 (37.29, 18.7088) -> (37.0431, 18.7088) construction
  line L3818 (37.0431, 18.7088) -> (36.843, 18.5087) construction
  line L3819 (36.843, 18.5087) -> (36.843, 18.2619) construction
  spline S1198 degree 3 poles (36.843, 18.2619) (36.843, 18.0151) (37.0431, 17.8149) (37.29, 17.8149) knots 0 0 0 0 1 1 1 1
  line L3820 (36.843, 18.2619) -> (36.843, 18.0151) construction
  line L3821 (36.843, 18.0151) -> (37.0431, 17.8149) construction
  line L3822 (37.0431, 17.8149) -> (37.29, 17.8149) construction
  spline S1199 degree 3 poles (37.29, 17.8149) (37.5369, 17.8149) (37.737, 18.0151) (37.737, 18.2619) knots 0 0 0 0 1 1 1 1
  line L3823 (37.29, 17.8149) -> (37.5369, 17.8149) construction
  line L3824 (37.5369, 17.8149) -> (37.737, 18.0151) construction
  line L3825 (37.737, 18.0151) -> (37.737, 18.2619) construction
  spline S1200 degree 3 poles (35.1829, 20.816) (35.1829, 21.0628) (34.9826, 21.2629) (34.7358, 21.2629) knots 0 0 0 0 1 1 1 1
  line L3826 (35.1829, 20.816) -> (35.1829, 21.0628) construction
  line L3827 (35.1829, 21.0628) -> (34.9826, 21.2629) construction
  line L3828 (34.9826, 21.2629) -> (34.7358, 21.2629) construction
  spline S1201 degree 3 poles (34.7358, 21.2629) (34.4891, 21.2629) (34.289, 21.0628) (34.289, 20.816) knots 0 0 0 0 1 1 1 1
  line L3829 (34.7358, 21.2629) -> (34.4891, 21.2629) construction
  line L3830 (34.4891, 21.2629) -> (34.289, 21.0628) construction
  line L3831 (34.289, 21.0628) -> (34.289, 20.816) construction
  spline S1202 degree 3 poles (34.289, 20.816) (34.289, 20.5692) (34.4891, 20.369) (34.7358, 20.369) knots 0 0 0 0 1 1 1 1
  line L3832 (34.289, 20.816) -> (34.289, 20.5692) construction
  line L3833 (34.289, 20.5692) -> (34.4891, 20.369) construction
  line L3834 (34.4891, 20.369) -> (34.7358, 20.369) construction
  spline S1203 degree 3 poles (34.7358, 20.369) (34.9826, 20.369) (35.1829, 20.5692) (35.1829, 20.816) knots 0 0 0 0 1 1 1 1
  line L3835 (34.7358, 20.369) -> (34.9826, 20.369) construction
  line L3836 (34.9826, 20.369) -> (35.1829, 20.5692) construction
  line L3837 (35.1829, 20.5692) -> (35.1829, 20.816) construction
  spline S1204 degree 3 poles (35.1829, 23.3701) (35.1829, 23.6169) (34.9826, 23.817) (34.7358, 23.817) knots 0 0 0 0 1 1 1 1
  line L3838 (35.1829, 23.3701) -> (35.1829, 23.6169) construction
  line L3839 (35.1829, 23.6169) -> (34.9826, 23.817) construction
  line L3840 (34.9826, 23.817) -> (34.7358, 23.817) construction
  spline S1205 degree 3 poles (34.7358, 23.817) (34.4891, 23.817) (34.289, 23.6169) (34.289, 23.3701) knots 0 0 0 0 1 1 1 1
  line L3841 (34.7358, 23.817) -> (34.4891, 23.817) construction
  line L3842 (34.4891, 23.817) -> (34.289, 23.6169) construction
  line L3843 (34.289, 23.6169) -> (34.289, 23.3701) construction
  spline S1206 degree 3 poles (34.289, 23.3701) (34.289, 23.1233) (34.4891, 22.9231) (34.7358, 22.9231) knots 0 0 0 0 1 1 1 1